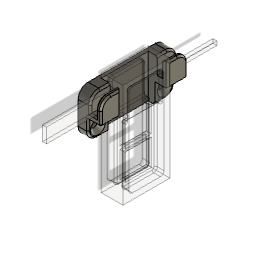
model (Autodesk Fusion 360 design; units mm, degrees)
Autodesk Fusion 360 part; units mm, degrees
note: some values were not read from the file. Chosen so that the rebuilt part matches the saved one: which face or edge a step refers to.
sketch "Sketch1" plane through (0, 0, 0) normal (0, 1, 0) x (1, 0, 0) in component "square"
  line L0 (0, 0) -> (28.3, 0)
  line L1 (28.3, 0) -> (28.3, -62.5)
  line L2 (28.3, -62.5) -> (0, -62.5)
  line L3 (0, -62.5) -> (0, 0)
  line L4 (0, -12.8) -> (-33.6, -12.8)
  line L5 (-33.6, -12.8) -> (-33.6, -10.4)
  line L6 (-33.6, -10.4) -> (0, -10.4)
  line L7 (28.3, -12.8) -> (69.1, -12.8)
  line L8 (69.1, -12.8) -> (69.1, -4)
  line L9 (69.1, -4) -> (28.3, -4)
  line L10 (3.6, -3.6) -> (24.7, -3.6)
  line L11 (24.7, -3.6) -> (24.7, -58.9)
  line L12 (24.7, -58.9) -> (3.6, -58.9)
  line L13 (3.6, -58.9) -> (3.6, -3.6)
  line L14 (7.2, -55.3) -> (21.1, -55.3)
  line L15 (21.1, -55.3) -> (21.1, -41.4)
  line L16 (21.1, -41.4) -> (7.2, -41.4)
  line L17 (7.2, -41.4) -> (7.2, -55.3)
  line L18 (14.15, -55.3) -> (14.15, -58.9) construction
  line L19 (21.1, -48.35) -> (24.7, -48.35) construction
  line L20 (7.2, -37.8) -> (21.1, -37.8)
  line L21 (21.1, -37.8) -> (21.1, -22.3)
  line L22 (21.1, -22.3) -> (7.2, -22.3)
  line L23 (7.2, -22.3) -> (7.2, -37.8)
  line L24 (14.15, -37.8) -> (14.15, -41.4) construction
  line L25 (7.2, -22.3) -> (3.6, -22.3)
  line L26 (21.1, -22.3) -> (24.7, -22.3)
  dimension "d1" = 28.3
  dimension "d2" = 62.5
  dimension "d3" = 8.8
  dimension "d4" = 2.4
  dimension "d5" = 10.4
  dimension "d6" = 4
  dimension "d7" = 40.8
  dimension "d8" = 33.6
  dimension "d9" = 3.6
  dimension "d10" = 3.6
  dimension "d11" = 18.7
  constraint horizontal L0
  constraint vertical L1
  constraint horizontal L2
  constraint vertical L3
  constraint coincident L0.start L3.end
  constraint horizontal L4
  constraint vertical L5
  constraint horizontal L6
  constraint coincident L3 L4.start
  constraint horizontal L7
  constraint vertical L8
  constraint horizontal L9
  constraint coincident L1 L7.start
  constraint coincident L3 L6.end
  constraint coincident L1 L9.end
  constraint collinear L4 L7
  constraint horizontal L14
  constraint vertical L15
  constraint horizontal L16
  constraint vertical L17
  constraint equal L14 L15
  constraint midpoint L14 L18.start
  constraint midpoint L12 L18.end
  constraint perpendicular L12 L18
  constraint midpoint L15 L19.start
  constraint coincident L11 L19.end
  constraint perpendicular L11 L19
  constraint equal L18 L19
  constraint horizontal L20
  constraint vertical L21
  constraint horizontal L22
  constraint vertical L23
  constraint collinear L17 L23
  constraint collinear L15 L21
  constraint midpoint L20 L24.start
  constraint midpoint L16 L24.end
  constraint equal L18 L24
  constraint coincident L13 L25.end
  constraint perpendicular L13 L25
  constraint coincident L11 L26.end
  constraint perpendicular L11 L26
  measures "d1" distance of L1.end L2.end
  measures "d2" distance of L0.start L2.end
  measures "d3" distance of L7.end L8.end
  measures "d4" distance of L4.end L5.end
  measures "d5" vertical distance of L0.start L5.end
  measures "d6" vertical distance of L0.end L8.end
  measures "d7" horizontal distance of L0.end L8.end
  measures "d8" horizontal distance of L0.start L5.end
  measures "d10" distance of L19.start L19.end
  measures "d11" vertical distance of L10.start L22.end
extrude "Extrude1" add sketch "Sketch1" along normal mid plane 13 contours L0 L1 L2 L3 makes body 1 in component "square"
extrude "Extrude2" add sketch "Sketch1" along normal mid plane 9 contours L10 L11 L13 L22 L25 L26 bodies 1 in component "square"
extrude "Extrude3" add sketch "Sketch1" along normal mid plane 3 contours L11 L12 L13 L20 L21 L23 L25 L26 bodies 1 in component "square"
extrude "Extrude4" add sketch "Sketch1" along normal mid plane 2.4 separate body contours L3 L4 L5 L6 | L1 L7 L8 L9 makes body 2 at (-11.2, 0.4, 12.8) makes body 3 at (55.5, 1.2, 9.8667) in component "square"
fillet "Fillet1" radius 2.1 8 edges at (3.6, -4, 58.9) (24.7, -4, 58.9) (3.6, -5.5, 3.6) (24.7, -5.5, 3.6) (24.7, 5.5, 3.6) (3.6, 5.5, 3.6) (24.7, 4, 58.9) (3.6, 4, 58.9) on bodies 1 in component "square"
fillet "Fillet2" radius 1 10 edges at (3.6, 4.5, 14) (4.2151, 4.5, 4.2151) (14.15, 4.5, 3.6) (24.0849, 4.5, 4.2151) (24.7, 4.5, 14) (24.7, -4.5, 14) (24.0849, -4.5, 4.2151) (14.15, -4.5, 3.6) (4.2151, -4.5, 4.2151) (3.6, -4.5, 14) 3 faces at (11.8333, 3.5, 22.3) (4.8, -1.5, 38.9667) (4.8, 1.5, 38.9667) on bodies 1 in component "square"
move_body "Move1" bodies 1 2 3 to x (1, 0, 0) y (0, -1, 0) z (0, 0, -1) at (0, 0, 0) in component "square"
sketch "Sketch1 (2)" plane through (0, 0, 0) normal (0, 0, 1) x (-1, 0, 0) in component "mount"
  line L0 (0, -6.5) -> (0, 6.5)
  line L1 (0, 6.5) -> (-28.3, 6.5)
  line L2 (-28.3, 6.5) -> (-28.3, -6.5)
  line L3 (-28.3, -6.5) -> (0, -6.5)
  line L4 (-69.1, 1.2) -> (33.6, 1.2)
  line L5 (33.6, 1.2) -> (33.6, -1.2)
  line L6 (33.6, -1.2) -> (-69.1, -1.2)
  line L7 (-69.1, -1.2) -> (-69.1, 1.2)
  line L8 (-40.3, 8.5) -> (12, 8.5)
  line L9 (12, 8.5) -> (12, -5.2)
  line L10 (12, -5.2) -> (-40.3, -5.2)
  line L11 (-40.3, -5.2) -> (-40.3, 8.5)
  line L12 (-14.15, -6.5) -> (-14.15, -5.2) construction
  line L13 (-40.3, 2.5) -> (12, 2.5)
  point P0 (-69.1, 1.2)
  point P1 (33.6, -1.2)
  dimension "d29" = 2
  dimension "d30" = 4
  dimension "d31" = 12
  dimension "d38" = 6
  constraint horizontal L4
  constraint vertical L5
  constraint horizontal L6
  constraint vertical L7
  constraint coincident P1 L5.end
  constraint coincident P0 L4.start
  constraint horizontal L8
  constraint vertical L9
  constraint horizontal L10
  constraint vertical L11
  constraint midpoint L3 L12.start
  constraint midpoint L10 L12.end
  constraint vertical L12
  constraint coincident L11 L13.start
  constraint coincident L9 L13.end
  constraint horizontal L13
  measures "d29" vertical distance of L1.end L8.start
  measures "d30" vertical distance of L6.end L10.end
  measures "d31" horizontal distance of L2.end L10.end
  measures "d38" distance of L8.end L13.end
extrude "Extrude1'" add sketch "Sketch1 (2)" against normal blind 4 from surface at -12.8 separate body contours L0 L6 L9 L10 | L0 L4 L6 L9 | L2 L6 L10 L11 | L0 L4 L9 L13 | L2 L4 L6 L11 | L0 L1 L2 L8 L9 L11 L13 | L2 L4 L11 L13 makes body 4 in component "mount"
extrude "Extrude2'" add sketch "Sketch1 (2)" along normal blind 10 from surface at -12.8 contours L0 L6 L9 L10 | L2 L6 L10 L11 | L0 L4 L9 L13 | L0 L1 L2 L8 L9 L11 L13 | L2 L4 L11 L13 bodies 4 in component "mount"
extrude "Extrude3'" add sketch "Sketch1 (2)" against normal blind 12 from surface at -16.8 contours L0 L1 L2 L8 L9 L11 L13 bodies 4 in component "mount"
sketch "Sketch2" plane through (0, -8.5, 0) normal (0, -1, 0) x (1, 0, 0) in component "mount"
  line L0 (-12, -2.8) -> (-12, -28.8)
  line L1 (-12, -28.8) -> (40.3, -28.8)
  line L2 (40.3, -28.8) -> (40.3, -2.8)
  line L3 (40.3, -2.8) -> (-12, -2.8)
  line L4 (-12, -16.8) -> (0, -16.8) construction
  line L5 (0, -16.8) -> (0, -28.8) construction
  line L6 (28.3, -28.8) -> (28.3, -16.8) construction
  line L7 (28.3, -16.8) -> (40.3, -16.8) construction
  circle A0 centre (-6, -22.8) radius 2
  circle A1 centre (34.3, -22.8) radius 2
  line L8 (-6, -16.8) -> (-6, -22.8) construction
  line L9 (-6, -22.8) -> (0, -22.8) construction
  line L10 (34.3, -16.8) -> (34.3, -22.8) construction
  line L11 (34.3, -22.8) -> (28.3, -22.8) construction
  point P0 (28.3, -16.8)
  point P1 (0, -16.8)
  dimension "d42" = 4
  constraint coincident L0 L4.start
  constraint coincident P1 L4.end
  constraint coincident L1 L5.end
  constraint coincident L1 L6.start
  constraint coincident P0 L6.end
  constraint coincident L2 L7.end
  constraint horizontal L7
  constraint horizontal L4
  constraint vertical L5
  constraint vertical L6
  constraint equal A0 A1
  constraint midpoint L4 L8.start
  constraint coincident A0.centre L8.end
  constraint midpoint L5 L9.end
  constraint midpoint L7 L10.start
  constraint coincident A1.centre L10.end
  constraint coincident L6 L11.end
  constraint parallel L9 L11
  constraint midpoint L6 L11.end
  constraint horizontal L11
  constraint vertical L10
  constraint vertical L8
  measures "d42" diameter of A0
extrude "Extrude4'" cut sketch "Sketch2" against normal blind 40 contours A0 | A1 bodies 4 in component "mount"
chamfer "Chamfer1" distance 2.5 angle 45 2 edges at (32.4353, -2.5, -23.5232) (-7.8647, -2.5, -23.5232) on bodies 4 in component "mount"
fillet "Fillet1'" radius 6 6 edges at (40.3, -5.5, -28.8) (-12, -5.5, -28.8) (40.3, 3.2, -2.8) (40.3, -4.85, -2.8) (-12, -4.85, -2.8) (-12, 3.2, -2.8) on bodies 4 in component "mount"
move_face "OffsetFaces1" offset -1 2 faces at (-6, 1.2, -8.1333) (34.3, 1.2, -8.1333) on bodies 4 in component "mount"
chamfer "Chamfer2" distance 1 angle 45 32 edges at (-3, -2.5, -28.8) (-10.2426, -2.5, -27.0426) (-12, -2.5, -19.8) (31.3, -2.5, -28.8) (0, 5.2, -9.8) (-12, 1.35, -16.8) (-12, 5.2, -12.8) (-12, 2.2, -10.8) (-12, 0.5, -12.8) (-12, -1.2, -10.8) (-6, 5.2, -16.8) (40.3, -2.5, -19.8) (38.5426, -2.5, -27.0426) (28.3, 5.2, -9.8) (31.3, -1.2, -2.8) (-3, -1.2, -2.8) (-10.2426, -1.2, -4.5574) (-10.2426, 2.2, -4.5574) (-3, 2.2, -2.8) (-3, 5.2, -2.8) (-10.2426, 5.2, -4.5574) (40.3, 1.35, -16.8) (40.3, -1.2, -10.8) (40.3, 0.5, -12.8) (40.3, 2.2, -10.8) (40.3, 5.2, -12.8) (34.3, 5.2, -16.8) (38.5426, 5.2, -4.5574) (31.3, 5.2, -2.8) (31.3, 2.2, -2.8) (38.5426, 2.2, -4.5574) (38.5426, -1.2, -4.5574) on bodies 4 in component "mount"
component "square" placed x (1, 0, 0) y (0, 1, 0) z (0, 0, 1) at (0, 0, 0)
component "mount" placed x (1, 0, 0) y (0, 1, 0) z (0, 0, 1) at (0, 0, 0)
equation "d10 = d9"
